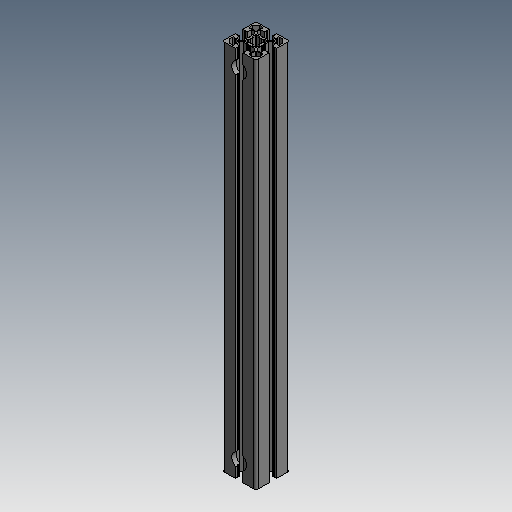
# Autodesk Inventor part: EFSB8-4545-500-LSV-RSV
Saved by Autodesk Inventor 2020 (Build 240168000, 168)
## iProperties
Part Number: EFSB8-4545-500-LSV-RSV
Material: 一般
Catalog Web Link: www.cadenas.de
Description: NEFS8-4545, EFS8-4545, EFSB8-4545, HFS8-4545, HFSB8-4545, CAF8-4545, NFSL8-4545, HFSL8-4545, GFS8-4545, HFSY8-4545-Aluminum Frames -8-45 Series-1 Row Groove 45 mm Square-Specified Length
Vendor: MISUMI
Document SubType Name: Modeling
Designer: partserver
Manufacturer: MISUMI
Mass: 354.547 g
Surface Area: 2824.45 cm^2
Volume: 354.547 cm^3
Density: 1 g/cm^3
Appearance: PSOLRGB-175-175-175
Category: PARTsolutions
Company: MISUMI
PSOL_IDENT_0: {$CADENAS_DATA\23d-libs\misumi\metric\38_al_extrusions_blackets\8_45\hfs8_4545.prj},668 {VTYP=3D},{N
PSOL_IDENT_1: B=EFSB8-4545-500-LSV-RSV},{LINA=EFSB8-4545-500-LSV-RSV},{NN=NEFS8-4545, EFS8-4545, EFSB8-4545, HFS8-
PSOL_IDENT_2: 4545, HFSB8-4545, CAF8-4545, NFSL8-4545, HFSL8-4545, GFS8-4545, HFSY8-4545},{DATE=23.09.2021 07:59:2
PSOL_IDENT_3: 2},{GEOMDATE=23.09.2021 07:56:34},{VERSION=},{LINEID=170},{WBVAR=L,ALT1,ALT2,ALT4,ALT5,CP5,DL5,DR5,A
PSOL_IDENT_4: LT6,ALT9,ALT10,ALT11,HP6,NHL6,DL6,NHR6,DR6,ALT7,ALT8,NH9,AH,BH,CH,DH,EH,NH10,AV,BV,CV,DV,EV,NH11,AP,
PSOL_IDENT_5: BP,CP,DP,EP,ALT12,ALT13,Z,NH12,XA,XB,XC,XD,XE,NH13,YA,YB,YC,YD,YE,ALT14,HP14,DL14,DR14,ALT15,HP15,DL
PSOL_IDENT_6: 15,DR15,ALT16,HP16,DL16,DR16,ALT19,ALT20},{WBNUMERIC=L,NH9,AH,BH,CH,DH,EH,NH10,AV,BV,CV,DV,EV,NH11,A
PSOL_IDENT_7: P,BP,CP,DP,EP,NH12,XA,XB,XC,XD,XE,NH13,YA,YB,YC,YD,YE}  {NB=EFSB8-4545-500-LSV-RSV},{LINA=EFSB8-4545
PSOL_IDENT_8: -500-LSV-RSV},{KT=DUMMY},{PN=EFSB8-4545-500-LSV-RSV},{TPS=EFSB8-4545},{MAT=A6N01SS-T5 Aluminum Alloy
PSOL_IDENT_9: },{ST=Black Anodize},{FRMW=45},{FRMH=45},{FRD=12.5},{L=500},{MASS=1.93},{SA=713},{LX=15.42x10^4},{LY=
PSOL_IDENT_10: 15.42x10^4},{ALT1=},{M1=0},{IDM1=10.106},{DPL1=0},{DPR1=0},{ALT1PN=},{ALT2=},{ALT2ALG= '','w/o End T
PSOL_IDENT_11: apping (Insert)','LHP','with LHP (Tapping on the Left (Insert))','RHP','with RHP (Tapping on the Rig
PSOL_IDENT_12: ht (Insert))','HPW','with HPW (Tapping on Both Ends (Insert))' },{M2=0},{DP2=0},{ALT2PN=},{ALT4=},{A
PSOL_IDENT_13: LT4ALG= '', 'w/o SC (High Precision Cut)', 'SC', 'with SC (High Precision Cut)' },{ALT4PN=},{ALT5=},
PSOL_IDENT_14: {ALT5ALG= '','w/o 45 Degree Cut','1','with 45 Degree Cut' },{CP5=},{CP5ALG= '','N/A' },{DL5=},{DL5AL
PSOL_IDENT_15: G= '','N/A' },{DR5=},{DR5ALG= '','N/A' },{FRMLALT5=0},{FRMRALT5=0},{ALT5PN=},{ALT6=},{ALT6ALG= '','w
PSOL_IDENT_16: /o Fastening Location Wrench Access Hole Alterations','1','with Fastening Location Wrench Access Hol
PSOL_IDENT_17: e Alterations' },{ALT9=},{ALT9ALG= '','w/o Location Specified Wrench Access Hole Alteratons (Horizon
PSOL_IDENT_18: tal)','1','with Location Specified Wrench Access Hole Alteratons (Horizontal)' },{ALT10=},{ALT10ALG=
PSOL_IDENT_19: '','w/o Location Specified Wrench Access Hole Alteratons (Vertical)','1','with Location Specified W
PSOL_IDENT_20: rench Access Hole Alteratons (Vertical)' },{ALT11=},{ALT11ALG= '','w/o Location Specified Wrench Acc
PSOL_IDENT_21: ess Hole Alteratons (Crisscross)','1','with Location Specified Wrench Access Hole Alteratons (Crissc
PSOL_IDENT_22: ross)' },{HP6=},{HP6ALG= '','N/A' },{NHL6=},{NHL6ALG= '','N/A' },{DL6=},{DL6ALG= '','N/A' },{NHR6=},
PSOL_IDENT_23: {NHR6ALG= '','N/A' },{DR6=},{DR6ALG= '','N/A' },{HL6=0.0},{HL6D=0.0},{HR6=0.0},{HR6D=0.0},{J6=0},{J6
PSOL_IDENT_24: D=0},{K6=0},{K6D=0},{DD6=0},{DD6ALG=0},{ALT7=},{ALT7ALG= '','N/A' },{ALT8=},{ALT8ALG= '','N/A' },{AL
PSOL_IDENT_25: T678PN=},{NH9=0},{NH9MAX=5},{NH9ALG=[0]},{AH=0.0},{AHMIN=7},{AHMAX=495},{AHALG=[0]},{BH=0.0},{BHMIN=
PSOL_IDENT_26: 2},{BHMAX=497},{BHALG=[0]},{CH=0.0},{CHMIN=2},{CHMAX=499},{CHALG=[0]},{DH=0.0},{DHMIN=2},{DHMAX=501}
PSOL_IDENT_27: ,{DHALG=[0]},{EH=0.0},{EHMIN=2},{EHMAX=493},{EHALG=[0]},{NH10=0},{NH10MAX=5},{NH10ALG=[0]},{AV=0.0},
PSOL_IDENT_28: {AVMIN=7},{AVMAX=495},{AVALG=[0]},{BV=0.0},{BVMIN=2},{BVMAX=497},{BVALG=[0]},{CV=0.0},{CVMIN=2},{CVM
PSOL_IDENT_29: AX=499},{CVALG=[0]},{DV=0.0},{DVMIN=2},{DVMAX=501},{DVALG=[0]},{EV=0.0},{EVMIN=2},{EVMAX=493},{EVALG=
PSOL_IDENT_30: [0]},{NH11=0},{NH11MAX=5},{NH11ALG=[0]},{AP=0.0},{APMIN=7},{APMAX=495},{APALG=[0]},{BP=0.0},{BPMIN=2
PSOL_IDENT_31: },{BPMAX=497},{BPALG=[0]},{CP=0.0},{CPMIN=2},{CPMAX=499},{CPALG=[0]},{DP=0.0},{DPMIN=2},{DPMAX=501},
PSOL_IDENT_32: {DPALG=[0]},{EP=0.0},{EPMIN=2},{EPMAX=493},{EPALG=[0]},{ALT9PN=},{ALT10PN=},{ALT11PN=},{ALT91011PN=}
PSOL_IDENT_33: ,{ALT12=},{ALT12ALG= '','w/o Counterbore Hole in Specified Position (Vertical)','1','with Counterbor
PSOL_IDENT_34: e Hole in Specified Position (Vertical)' },{ALT13=},{ALT13ALG= '','w/o Counterbore Hole in Specified
PSOL_IDENT_35: Position (Horizontal)','1','with Counterbore Hole in Specified Position (Horizontal)' },{Z=},{ZALG=
PSOL_IDENT_36: '','N/A' },{DD12=0.0},{DD112=0},{NH12=0},{NH12MAX=5},{NH12ALG=[0]},{XA=0.0},{XAMIN=7},{XAMAX=495},{
PSOL_IDENT_37: XAALG=[0]},{XB=0.0},{XBMIN=2},{XBMAX=497},{XBALG=[0]},{XC=0.0},{XCMIN=2},{XCMAX=499},{XCALG=[0]},{XD=
PSOL_IDENT_38: 0.0},{XDMIN=2},{XDMAX=501},{XDALG=[0]},{XE=0.0},{XEMIN=2},{XEMAX=493},{XEALG=[0]},{NH13=0},{NH13MAX=
PSOL_IDENT_39: 5},{NH13ALG=[0]},{YA=0.0},{YAMIN=7},{YAMAX=495},{YAALG=[0]},{YB=0.0},{YBMIN=2},{YBMAX=497},{YBALG=[0
PSOL_IDENT_40: ]},{YC=0.0},{YCMIN=2},{YCMAX=499},{YCALG=[0]},{YD=0.0},{YDMIN=2},{YDMAX=501},{YDALG=[0]},{YE=0.0},{Y
PSOL_IDENT_41: EMIN=2},{YEMAX=493},{YEALG=[0]},{ALT12133D=13.000},{ALT12PN=},{ALT13PN=},{ALT1213PN=},{ALT14=},{ALT1
PSOL_IDENT_42: 4ALG= '','w/o D Type Hole Alteration','1','with D Type Hole Alteration' },{HP14=},{HP14ALG= '','N/A'
PSOL_IDENT_43: },{DL14=},{DL14ALG= '','N/A' },{DR14=},{DR14ALG= '','N/A' },{H14=0.0},{D14=0.0},{ALT14PN=},{ALT15=1
PSOL_IDENT_44: },{ALT15ALG= '','w/o S Type Hole Alteration','1','with S Type Hole Alteration' },{HP15=LR},{HP15ALG=
PSOL_IDENT_45: 'L','Left','R','Right','LR','Both Sides' },{DL15=V},{DL15ALG= 'H','Horizontal','V','Vertical','P','
PSOL_IDENT_46: Crisscross' },{DR15=V},{DR15ALG= 'H','Horizontal','V','Vertical','P','Crisscross' },{H15=22.5},{D115=
PSOL_IDENT_47: 20},{D215=15.1},{ALT15PN=-LSV-RSV},{ALT16=},{ALT16ALG= '','w/o M Type Hole Alteration','1','with M T
PSOL_IDENT_48: ype Hole Alteration' },{HP16=},{HP16ALG= '','N/A' },{DL16=},{DL16ALG= '','N/A' },{DR16=},{DR16ALG= ''
PSOL_IDENT_49: ,'N/A' },{H116=0.0},{D16=0.0},{ALT16PN=},{ALT19=},{ALT19ALG= '','N/A' },{M19=0},{DP19=0},{ALT19PN=},
PSOL_IDENT_50: {ALT20=},{ALT20PN=},{ERRORALT01=OK},{ERRORALT02=OK},{ERRORALT05=OK},{ERRORALT06091=OK},{ERRORALT0609
PSOL_IDENT_51: 2=OK},{ERRORALT06093=OK},{ERRORALT06094=OK},{ERRORALT06101=OK},{ERRORALT06102=OK},{ERRORALT06103=OK}
PSOL_IDENT_52: ,{ERRORALT06104=OK},{ERRORALT06111=OK},{ERRORALT06112=OK},{ERRORALT06113=OK},{ERRORALT06114=OK},{ERR
PSOL_IDENT_53: ORALT06121=OK},{ERRORALT06122=OK},{ERRORALT06123=OK},{ERRORALT06124=OK},{ERRORALT06131=OK},{ERRORALT
PSOL_IDENT_54: 06132=OK},{ERRORALT06133=OK},{ERRORALT06134=OK},{ERRORALT0614=OK},{ERRORALT0615=OK},{ERRORALT0616=OK
PSOL_IDENT_55: },{ERRORALT0619=OK},{ERRORALT0911=OK},{ERRORALT0913=OK},{ERRORALT0914=OK},{ERRORALT0915=OK},{ERRORAL
PSOL_IDENT_56: T0916=OK},{ERRORALT0919=OK},{ERRORALT1011=OK},{ERRORALT1012=OK},{ERRORALT1014=OK},{ERRORALT1015=OK},
PSOL_IDENT_57: {ERRORALT1016=OK},{ERRORALT1019=OK},{ERRORALT1112=OK},{ERRORALT1113=OK},{ERRORALT1114=OK},{ERRORALT1
PSOL_IDENT_58: 115=OK},{ERRORALT1116=OK},{ERRORALT1119=OK},{ERRORALT1214=OK},{ERRORALT1215=OK},{ERRORALT1216=OK},{E
PSOL_IDENT_59: RRORALT1219=OK},{ERRORALT1314=OK},{ERRORALT1315=OK},{ERRORALT1316=OK},{ERRORALT1319=OK},{ERRORALT141
PSOL_IDENT_60: 5=OK},{ERRORALT1416=OK},{ERRORALT1419=OK},{ERRORALT1516=OK},{ERRORALT1519=OK},{ERRORALT1619=OK},{ERR
PSOL_IDENT_61: ORPN=},{COLOR=}
NB: EFSB8-4545-500-LSV-RSV
NN: NEFS8-4545, EFS8-4545, EFSB8-4545, HFS8-4545, HFSB8-4545, CAF8-4545, NFSL8-4545, HFSL8-4545, GFS8-4545, HFSY8-4545
NT: Aluminum Frames -8-45 Series-1 Row Groove 45 mm Square-Specified Length
NBSYN: $PN.
LINA: EFSB8-4545-500-LSV-RSV
CATALOG: Misumi
PN: EFSB8-4545-500-LSV-RSV
TPS: EFSB8-4545
MAT: A6N01SS-T5 Aluminum Alloy
ST: Black Anodize
L: 500
MASS: 1.93
SA: 713
LX: 15.42x10^4
LY: 15.42x10^4
ALT1: w/o End Tapping
M1: 0
DPL1: 0
DPR1: 0
ALT2: w/o End Tapping (Insert)
M2: 0
DP2: 0
ALT4: w/o SC (High Precision Cut)
ALT5: w/o 45 Degree Cut
CP5: N/A
DL5: N/A
DR5: N/A
ALT6: w/o Fastening Location Wrench Access Hole Alterations
ALT9: w/o Location Specified Wrench Access Hole Alteratons (Horizontal)
ALT10: w/o Location Specified Wrench Access Hole Alteratons (Vertical)
ALT11: w/o Location Specified Wrench Access Hole Alteratons (Crisscross)
HP6: N/A
NHL6: N/A
DL6: N/A
NHR6: N/A
DR6: N/A
HL6D: 0
HR6D: 0
J6D: 0
K6D: 0
DD6: 0
ALT7: N/A
ALT8: N/A
NH9: 0
AH: 0
BH: 0
CH: 0
DH: 0
EH: 0
NH10: 0
AV: 0
BV: 0
CV: 0
DV: 0
EV: 0
NH11: 0
AP: 0
BP: 0
CP: 0
DP: 0
EP: 0
ALT12: w/o Counterbore Hole in Specified Position (Vertical)
ALT13: w/o Counterbore Hole in Specified Position (Horizontal)
Z: N/A
DD12: 0
DD112: 0
NH12: 0
XA: 0
XB: 0
XC: 0
XD: 0
XE: 0
NH13: 0
YA: 0
YB: 0
YC: 0
YD: 0
YE: 0
ALT14: w/o D Type Hole Alteration
HP14: N/A
DL14: N/A
DR14: N/A
H14: 0
D14: 0
ALT15: with S Type Hole Alteration
HP15: Both Sides
DL15: Vertical
DR15: Vertical
H15: 22.5
D115: 20
D215: 15.1
ALT16: w/o M Type Hole Alteration
HP16: N/A
DL16: N/A
DR16: N/A
H116: 0
D16: 0
ALT19: N/A
M19: 0
DP19: 0
ALT20: w/o CW (End Face C Chamfering)
SUPPLIER: MISUMI
ARTICLENO: EFSB8-4545-500-LSV-RSV
BOMINFO: EFSB8-4545-500-LSV-RSV
CREATOR: CADENAS GmbH
Title: EFSB8-4545-500-LSV-RSV
Author: Cadenas PARTsolutions
Comments: Aluminum Frames -8-45 Series-1 Row Groove 45 mm Square-Specified Length
Autodesk Inventor part; units mm, degrees
ref_plane "YZ Plane" through (0, 0, 0) normal (1, 0, 0) x (0, 1, 0)
ref_plane "XZ Plane" through (0, 0, 0) normal (0, 1, 0) x (-1, 0, 0)
ref_plane "XY Plane" through (0, 0, 0) normal (0, 0, 1) x (1, 0, 0)
sketch "Sketch_73" plane through (0, 0, 0) normal (0, 0, 1) x (1, 0, 0)
  arc A0 (-22.5, -19.5) -> (-19.5, -22.5) centre (-19.5, -19.5) ccw
  line L0 (-19.5, -22.5) -> (-5, -22.5)
  line L1 (-5, -22.5) -> (-5, -20.366)
  arc A1 (-5, -18.634) -> (-5, -20.366) centre (-4.5, -19.5) ccw
  line L2 (-5, -18.634) -> (-5, -16.5)
  line L3 (-5, -16.5) -> (-10, -16.5)
  line L4 (-10, -16.5) -> (-10, -12.1213)
  line L5 (-10, -12.1213) -> (-7.3787, -9.5)
  line L6 (-7.3787, -9.5) -> (-2.6939, -9.5)
  line L7 (-2.6939, -9.5) -> (-1.7, -9.2887)
  line L8 (-1.7, -9.2887) -> (-0.7575, -9.4891)
  arc A2 (-0.7575, -9.4891) -> (-0.4036, -9.433) centre (-0.6536, -9) ccw
  line L9 (-0.4036, -9.433) -> (0, -9.2)
  line L10 (0, -9.2) -> (0.4036, -9.433)
  arc A3 (0.4036, -9.433) -> (0.7575, -9.4891) centre (0.6536, -9) ccw
  line L11 (0.7575, -9.4891) -> (1.7, -9.2887)
  line L12 (1.7, -9.2887) -> (2.6939, -9.5)
  line L13 (2.6939, -9.5) -> (7.3787, -9.5)
  line L14 (7.3787, -9.5) -> (10, -12.1213)
  line L15 (10, -12.1213) -> (10, -16.5)
  line L16 (10, -16.5) -> (5, -16.5)
  line L17 (5, -16.5) -> (5, -18.634)
  arc A4 (5, -20.366) -> (5, -18.634) centre (4.5, -19.5) ccw
  line L18 (5, -20.366) -> (5, -22.5)
  line L19 (5, -22.5) -> (19.5, -22.5)
  arc A5 (19.5, -22.5) -> (22.5, -19.5) centre (19.5, -19.5) ccw
  line L20 (22.5, -19.5) -> (22.5, -5)
  line L21 (22.5, -5) -> (20.366, -5)
  arc A6 (18.634, -5) -> (20.366, -5) centre (19.5, -4.5) ccw
  line L22 (18.634, -5) -> (16.5, -5)
  line L23 (16.5, -5) -> (16.5, -10)
  line L24 (16.5, -10) -> (12.1213, -10)
  line L25 (12.1213, -10) -> (9.5, -7.3787)
  line L26 (9.5, -7.3787) -> (9.5, -2.6939)
  line L27 (9.5, -2.6939) -> (9.2887, -1.7)
  line L28 (9.2887, -1.7) -> (9.4891, -0.7575)
  arc A7 (9.4891, -0.7575) -> (9.433, -0.4036) centre (9, -0.6536) ccw
  line L29 (9.433, -0.4036) -> (9.2, 0)
  line L30 (9.2, 0) -> (9.433, 0.4036)
  arc A8 (9.433, 0.4036) -> (9.4891, 0.7575) centre (9, 0.6536) ccw
  line L31 (9.4891, 0.7575) -> (9.2887, 1.7)
  line L32 (9.2887, 1.7) -> (9.5, 2.6939)
  line L33 (9.5, 2.6939) -> (9.5, 7.3787)
  line L34 (9.5, 7.3787) -> (12.1213, 10)
  line L35 (12.1213, 10) -> (16.5, 10)
  line L36 (16.5, 10) -> (16.5, 5)
  line L37 (16.5, 5) -> (18.634, 5)
  arc A9 (20.366, 5) -> (18.634, 5) centre (19.5, 4.5) ccw
  line L38 (20.366, 5) -> (22.5, 5)
  line L39 (22.5, 5) -> (22.5, 19.5)
  arc A10 (22.5, 19.5) -> (19.5, 22.5) centre (19.5, 19.5) ccw
  line L40 (19.5, 22.5) -> (5, 22.5)
  line L41 (5, 22.5) -> (5, 20.366)
  arc A11 (5, 18.634) -> (5, 20.366) centre (4.5, 19.5) ccw
  line L42 (5, 18.634) -> (5, 16.5)
  line L43 (5, 16.5) -> (10, 16.5)
  line L44 (10, 16.5) -> (10, 12.1213)
  line L45 (10, 12.1213) -> (7.3787, 9.5)
  line L46 (7.3787, 9.5) -> (2.6939, 9.5)
  line L47 (2.6939, 9.5) -> (1.7, 9.2887)
  line L48 (1.7, 9.2887) -> (0.7575, 9.4891)
  arc A12 (0.7575, 9.4891) -> (0.4036, 9.433) centre (0.6536, 9) ccw
  line L49 (0.4036, 9.433) -> (0, 9.2)
  line L50 (0, 9.2) -> (-0.4036, 9.433)
  arc A13 (-0.4036, 9.433) -> (-0.7575, 9.4891) centre (-0.6536, 9) ccw
  line L51 (-0.7575, 9.4891) -> (-1.7, 9.2887)
  line L52 (-1.7, 9.2887) -> (-2.6939, 9.5)
  line L53 (-2.6939, 9.5) -> (-7.3787, 9.5)
  line L54 (-7.3787, 9.5) -> (-10, 12.1213)
  line L55 (-10, 12.1213) -> (-10, 16.5)
  line L56 (-10, 16.5) -> (-5, 16.5)
  line L57 (-5, 16.5) -> (-5, 18.634)
  arc A14 (-5, 20.366) -> (-5, 18.634) centre (-4.5, 19.5) ccw
  line L58 (-5, 20.366) -> (-5, 22.5)
  line L59 (-5, 22.5) -> (-19.5, 22.5)
  arc A15 (-19.5, 22.5) -> (-22.5, 19.5) centre (-19.5, 19.5) ccw
  line L60 (-22.5, 19.5) -> (-22.5, 5)
  line L61 (-22.5, 5) -> (-20.366, 5)
  arc A16 (-18.634, 5) -> (-20.366, 5) centre (-19.5, 4.5) ccw
  line L62 (-18.634, 5) -> (-16.5, 5)
  line L63 (-16.5, 5) -> (-16.5, 10)
  line L64 (-16.5, 10) -> (-12.1213, 10)
  line L65 (-12.1213, 10) -> (-9.5, 7.3787)
  line L66 (-9.5, 7.3787) -> (-9.5, 2.6939)
  line L67 (-9.5, 2.6939) -> (-9.2887, 1.7)
  line L68 (-9.2887, 1.7) -> (-9.4891, 0.7575)
  arc A17 (-9.4891, 0.7575) -> (-9.433, 0.4036) centre (-9, 0.6536) ccw
  line L69 (-9.433, 0.4036) -> (-9.2, 0)
  line L70 (-9.2, 0) -> (-9.433, -0.4036)
  arc A18 (-9.433, -0.4036) -> (-9.4891, -0.7575) centre (-9, -0.6536) ccw
  line L71 (-9.4891, -0.7575) -> (-9.2887, -1.7)
  line L72 (-9.2887, -1.7) -> (-9.5, -2.6939)
  line L73 (-9.5, -2.6939) -> (-9.5, -7.3787)
  line L74 (-9.5, -7.3787) -> (-12.1213, -10)
  line L75 (-12.1213, -10) -> (-16.5, -10)
  line L76 (-16.5, -10) -> (-16.5, -5)
  line L77 (-16.5, -5) -> (-18.634, -5)
  arc A19 (-20.366, -5) -> (-18.634, -5) centre (-19.5, -4.5) ccw
  line L78 (-20.366, -5) -> (-22.5, -5)
  line L79 (-22.5, -5) -> (-22.5, -19.5)
  arc A20 (11.55, 20.5) -> (10.8, 17.701) centre (11.55, 19) ccw
  arc A21 (11.3, 16.8349) -> (10.8, 17.701) centre (10.3, 16.8349) ccw
  line L80 (11.3, 16.8349) -> (11.3, 11.8)
  arc A22 (11.3, 11.8) -> (11.8, 11.3) centre (11.8, 11.8) ccw
  line L81 (11.8, 11.3) -> (16.8349, 11.3)
  arc A23 (17.701, 10.8) -> (16.8349, 11.3) centre (16.8349, 10.3) ccw
  arc A24 (17.701, 10.8) -> (20.5, 11.55) centre (19, 11.55) ccw
  line L82 (20.5, 11.55) -> (20.5, 15.1482)
  arc A25 (20.5, 15.1482) -> (20.2071, 15.8553) centre (19.5, 15.1482) ccw
  line L83 (20.2071, 15.8553) -> (15.8553, 20.2071)
  arc A26 (15.8553, 20.2071) -> (15.1482, 20.5) centre (15.1482, 19.5) ccw
  line L84 (15.1482, 20.5) -> (11.55, 20.5)
  arc A27 (10.8, -17.701) -> (11.55, -20.5) centre (11.55, -19) ccw
  line L85 (11.55, -20.5) -> (15.1482, -20.5)
  arc A28 (15.1482, -20.5) -> (15.8553, -20.2071) centre (15.1482, -19.5) ccw
  line L86 (15.8553, -20.2071) -> (20.2071, -15.8553)
  arc A29 (20.2071, -15.8553) -> (20.5, -15.1482) centre (19.5, -15.1482) ccw
  line L87 (20.5, -15.1482) -> (20.5, -11.55)
  arc A30 (20.5, -11.55) -> (17.701, -10.8) centre (19, -11.55) ccw
  arc A31 (16.8349, -11.3) -> (17.701, -10.8) centre (16.8349, -10.3) ccw
  line L88 (16.8349, -11.3) -> (11.8, -11.3)
  arc A32 (11.8, -11.3) -> (11.3, -11.8) centre (11.8, -11.8) ccw
  line L89 (11.3, -11.8) -> (11.3, -16.8349)
  arc A33 (10.8, -17.701) -> (11.3, -16.8349) centre (10.3, -16.8349) ccw
  line L90 (-20.5, 15.1482) -> (-20.5, 11.55)
  arc A34 (-20.5, 11.55) -> (-17.701, 10.8) centre (-19, 11.55) ccw
  arc A35 (-16.8349, 11.3) -> (-17.701, 10.8) centre (-16.8349, 10.3) ccw
  line L91 (-16.8349, 11.3) -> (-11.8, 11.3)
  arc A36 (-11.8, 11.3) -> (-11.3, 11.8) centre (-11.8, 11.8) ccw
  line L92 (-11.3, 11.8) -> (-11.3, 16.8349)
  arc A37 (-10.8, 17.701) -> (-11.3, 16.8349) centre (-10.3, 16.8349) ccw
  arc A38 (-10.8, 17.701) -> (-11.55, 20.5) centre (-11.55, 19) ccw
  line L93 (-11.55, 20.5) -> (-15.1482, 20.5)
  arc A39 (-15.1482, 20.5) -> (-15.8553, 20.2071) centre (-15.1482, 19.5) ccw
  line L94 (-15.8553, 20.2071) -> (-20.2071, 15.8553)
  arc A40 (-20.2071, 15.8553) -> (-20.5, 15.1482) centre (-19.5, 15.1482) ccw
  arc A41 (-20.5, -15.1482) -> (-20.2071, -15.8553) centre (-19.5, -15.1482) ccw
  line L95 (-20.2071, -15.8553) -> (-15.8553, -20.2071)
  arc A42 (-15.8553, -20.2071) -> (-15.1482, -20.5) centre (-15.1482, -19.5) ccw
  line L96 (-15.1482, -20.5) -> (-11.55, -20.5)
  arc A43 (-11.55, -20.5) -> (-10.8, -17.701) centre (-11.55, -19) ccw
  arc A44 (-11.3, -16.8349) -> (-10.8, -17.701) centre (-10.3, -16.8349) ccw
  line L97 (-11.3, -16.8349) -> (-11.3, -11.8)
  arc A45 (-11.3, -11.8) -> (-11.8, -11.3) centre (-11.8, -11.8) ccw
  line L98 (-11.8, -11.3) -> (-16.8349, -11.3)
  arc A46 (-17.701, -10.8) -> (-16.8349, -11.3) centre (-16.8349, -10.3) ccw
  arc A47 (-17.701, -10.8) -> (-20.5, -11.55) centre (-19, -11.55) ccw
  line L99 (-20.5, -11.55) -> (-20.5, -15.1482)
  constraints: 200 end point, 96 point on circle, 48 centre point
extrude "Extrusion1" add sketch "Sketch_73" against normal blind 500
sketch "Sketch_91" plane through (0, 0, 0) normal (0, 0, 1) x (1, 0, 0)
  arc A0 (-7.9, -7.4) -> (-7.4, -7.9) centre (-7.4, -7.4) ccw
  line L0 (-7.4, -7.9) -> (-3.6, -7.9)
  arc A1 (-3.6, -7.9) -> (-3.0139, -7.1717) centre (-3.6, -7.3) ccw
  arc A2 (-1.756, -5.9982) -> (-3.0139, -7.1717) centre (-2.037, -6.958) ccw
  arc A3 (-1.756, -5.9982) -> (1.756, -5.9982) centre (0, 0) ccw
  arc A4 (3.0139, -7.1717) -> (1.756, -5.9982) centre (2.037, -6.958) ccw
  arc A5 (3.0139, -7.1717) -> (3.6, -7.9) centre (3.6, -7.3) ccw
  line L1 (3.6, -7.9) -> (7.4, -7.9)
  arc A6 (7.4, -7.9) -> (7.9, -7.4) centre (7.4, -7.4) ccw
  line L2 (7.9, -7.4) -> (7.9, -3.6)
  arc A7 (7.9, -3.6) -> (7.1717, -3.0139) centre (7.3, -3.6) ccw
  arc A8 (5.9982, -1.756) -> (7.1717, -3.0139) centre (6.958, -2.037) ccw
  arc A9 (5.9982, -1.756) -> (5.9982, 1.756) centre (0, 0) ccw
  arc A10 (7.1717, 3.0139) -> (5.9982, 1.756) centre (6.958, 2.037) ccw
  arc A11 (7.1717, 3.0139) -> (7.9, 3.6) centre (7.3, 3.6) ccw
  line L3 (7.9, 3.6) -> (7.9, 7.4)
  arc A12 (7.9, 7.4) -> (7.4, 7.9) centre (7.4, 7.4) ccw
  line L4 (7.4, 7.9) -> (3.6, 7.9)
  arc A13 (3.6, 7.9) -> (3.0139, 7.1717) centre (3.6, 7.3) ccw
  arc A14 (1.756, 5.9982) -> (3.0139, 7.1717) centre (2.037, 6.958) ccw
  arc A15 (1.756, 5.9982) -> (-1.756, 5.9982) centre (0, 0) ccw
  arc A16 (-3.0139, 7.1717) -> (-1.756, 5.9982) centre (-2.037, 6.958) ccw
  arc A17 (-3.0139, 7.1717) -> (-3.6, 7.9) centre (-3.6, 7.3) ccw
  line L5 (-3.6, 7.9) -> (-7.4, 7.9)
  arc A18 (-7.4, 7.9) -> (-7.9, 7.4) centre (-7.4, 7.4) ccw
  line L6 (-7.9, 7.4) -> (-7.9, 3.6)
  arc A19 (-7.9, 3.6) -> (-7.1717, 3.0139) centre (-7.3, 3.6) ccw
  arc A20 (-5.9982, 1.756) -> (-7.1717, 3.0139) centre (-6.958, 2.037) ccw
  arc A21 (-5.9982, 1.756) -> (-5.9982, -1.756) centre (0, 0) ccw
  arc A22 (-7.1717, -3.0139) -> (-5.9982, -1.756) centre (-6.958, -2.037) ccw
  arc A23 (-7.1717, -3.0139) -> (-7.9, -3.6) centre (-7.3, -3.6) ccw
  line L7 (-7.9, -3.6) -> (-7.9, -7.4)
  constraints: 48 point on circle, 24 centre point, 16 end point
extrude "Extrusion2" cut sketch "Sketch_91" against normal blind 500
sketch "Sketch_71" plane through (0, 0, 0) normal (1, 0, 0) x (0, 0, -1)
  line L0 (22.5, -22.5) -> (22.5, 22.5)
  line L1 (22.5, 22.5) -> (32.5, 22.5)
  line L2 (32.5, 22.5) -> (32.5, 16.5)
  line L3 (32.5, 16.5) -> (30.05, 16.5)
  line L4 (30.05, 16.5) -> (30.05, -16.5)
  line L5 (30.05, -16.5) -> (32.5, -16.5)
  line L6 (32.5, -16.5) -> (32.5, -22.5)
  line L7 (32.5, -22.5) -> (22.5, -22.5)
  line L8 (22.5, -22.5) -> (22.5, 22.5)
  constraints: 18 end point
revolve "Revolution1" cut sketch "Sketch_71" angle 360 about axis through (0, -22.5, -22.5) along (0, -1, 0)
sketch "Sketch_72" plane through (0, 0, 0) normal (1, 0, 0) x (0, 0, -1)
  line L0 (477.5, -22.5) -> (477.5, 22.5)
  line L1 (477.5, 22.5) -> (487.5, 22.5)
  line L2 (487.5, 22.5) -> (487.5, 16.5)
  line L3 (487.5, 16.5) -> (485.05, 16.5)
  line L4 (485.05, 16.5) -> (485.05, -16.5)
  line L5 (485.05, -16.5) -> (487.5, -16.5)
  line L6 (487.5, -16.5) -> (487.5, -22.5)
  line L7 (487.5, -22.5) -> (477.5, -22.5)
  line L8 (477.5, -22.5) -> (477.5, 22.5)
  constraints: 18 end point
revolve "Revolution2" cut sketch "Sketch_72" angle 360 about axis through (0, -22.5, -477.5) along (0, -1, 0)
ref_plane "C1_XY" through (0, 0, 0) normal (0, 0, 1) x (1, 0, 0)
ref_plane "C1_YZ" through (0, 0, 0) normal (1, 0, 0) x (0, 1, 0)
ref_plane "C1_ZX" through (0, 0, 0) normal (0, 1, 0) x (0, 0, 1)
body "Solid1"
